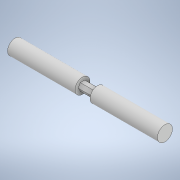
# Autodesk Inventor part: pin
Saved by Autodesk Inventor 2020 (Build 240168000, 168)
## iProperties
Created: 2020-01-14
Part Number: pin
Material: Generic
Document SubType Name: Modeling
Designer: woodn
Density: 1 g/cm^3
Appearance: Default
Author: woodn
Autodesk Inventor part; units mm, degrees
ref_plane "YZ Plane" through (0, 0, 0) normal (1, 0, 0) x (0, 1, 0)
ref_plane "XZ Plane" through (0, 0, 0) normal (0, 1, 0) x (-1, 0, 0)
ref_plane "XY Plane" through (0, 0, 0) normal (0, 0, 1) x (1, 0, 0)
sketch "Sketch1" plane through (0, 0, 0) normal (1, 0, 0) x (0, 1, 0)
  circle A0 centre (0, 0) radius 12.7
  dimension "d0" = 25.4
  constraints: 1 centre point, 1 coincident
  measures "d0" diameter of A0
extrude "Extrusion1" add sketch "Sketch1" against normal blind 254
sketch "Sketch2" plane through (0, 0, 0) normal (1, 0, 0) x (0, 0, -1)
  line L0 (3.6609, 6.353) -> (7.3323, 0.006)
  line L1 (7.3323, 0.006) -> (3.6714, -6.347)
  line L2 (3.6714, -6.347) -> (-3.6609, -6.353)
  line L3 (-3.6609, -6.353) -> (-7.3323, -0.006)
  line L4 (-7.3323, -0.006) -> (-3.6714, 6.347)
  line L5 (-3.6714, 6.347) -> (3.6609, 6.353)
  circle A0 centre (0, 0) radius 12.7
  dimension "d3" = 6.35
  constraints: 12 end point, 2 coincident, 1 centre point, 13 other
  measures "d3" distance from line of point (0, 0) L5
extrude "Extrusion2" cut sketch "Sketch2" against normal blind 254
extrude "Extrusion3" add sketch "Sketch2" against normal blind 114.3 contours L0 L1 L2 L3 L4 L5 | A0
sketch "Sketch3" plane through (-254, 0, 0) normal (-1, 0, 0) x (0, 0, 1)
  circle A0 centre (0, 0) radius 12.7 projected
  circle A1 centre (0, 0) radius 12.7
  constraints: 1 centre point, 1 coincident
extrude "Extrusion4" add sketch "Sketch3" against normal blind 114.3
body "Solid1"
